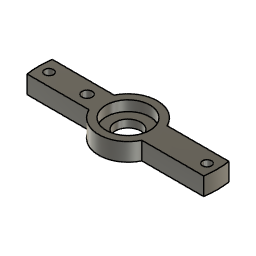
wind_speed_base (Autodesk Fusion 360 design; units mm, degrees)
Autodesk Fusion 360 part; units mm, degrees
note: some values were not read from the file. Set by a fixed rule: which sketch regions a step uses.
sketch "Szkic1" plane through (0, 0, 0) normal (0, 0, 1) x (1, 0, 0)
  circle A0 centre (0, 0) radius 11.5
  circle A1 centre (0, 0) radius 8.6
  circle A2 centre (0, 0) radius 5
  dimension "d1" = 23
  dimension "d2" = 17.2
  dimension "d7" = 10
  constraint coincident A0.centre A1.centre
  measures "d1" diameter of A0
  measures "d2" diameter of A1
  measures "d7" diameter of A2
extrude "Wyciągnięcie proste1" add sketch "Szkic1" along normal blind 7 contours A0
extrude "Wyciągnięcie proste2" add sketch "Szkic1" along normal blind 3 contours A1
sketch "Szkic2" plane through (0, 0, 0) normal (0, 0, 1) x (1, 0, 0)
  line L0 (20, -5) -> (-20, -5)
  line L1 (-20, 5) -> (20, 5)
  line L2 (20, -5) -> (-20, 5) construction
  line L3 (-20, -5) -> (20, 5) construction
  line L4 (35, -4.95) -> (-35, -4.95)
  line L5 (-35, -4.95) -> (-35, 4.95)
  line L6 (-35, 4.95) -> (35, 4.95)
  line L7 (35, 4.95) -> (35, -4.95)
  line L8 (35, -4.95) -> (-35, 4.95) construction
  line L9 (-20, -5) -> (-24, -5)
  line L10 (-24, 5) -> (-20, 5)
  circle A0 centre (0, 0) radius 11.5
  line L11 (-35, -4.95) -> (-11.3867, -1.6104) construction
  line L12 (0, 0) -> (35, 4.95) construction
  circle A1 centre (0, 0) radius 35
  circle A2 centre (-31, 0) radius 1.75
  circle A3 centre (31, 0) radius 1.75
  circle A4 centre (-15.9999, -0.05) radius 2
  dimension "d9" = 10
  dimension "d10" = 70
  dimension "d11" = 9.9
  dimension "d36" = 3.5
  dimension "d37" = 4
  dimension "d38" = 4
  dimension "d68" = 4
  dimension "d69" = 5
  dimension "d70" = 16
  constraint horizontal L0
  constraint parallel L0 L1
  constraint coincident L2 A0.centre
  constraint coincident L3 A0.centre
  constraint coincident A0.centre L12.start
  constraint horizontal L4
  constraint perpendicular L4 L5
  constraint parallel L4 L6
  constraint parallel L5 L7
  constraint coincident L8 A0.centre
  constraint coincident A0.centre L11
  constraint horizontal L9
  constraint horizontal L10
  constraint coincident A0 L11.end
  constraint collinear L11 L12
  constraint tangent L7 A1
  constraint horizontal A0.centre A3.centre
  constraint horizontal A0.centre A2.centre
  constraint equal A2 A3
  measures "d9" distance of L0.end L1.start
  measures "d10" distance of L5.end L6.end
  measures "d11" distance of L4.end L5.end
  measures "d36" diameter of A3
  measures "d37" distance of L7 A3.centre
  measures "d38" distance of L5 A2.centre
  measures "d68" diameter of A4
  measures "d69" distance of L6 A4.centre
  measures "d70" distance of A0.centre A4.centre
extrude "Wyciągnięcie proste3" add sketch "Szkic2" along normal blind 7 contours L4 L6 A0 A1 | L4 L6 A0 A1
